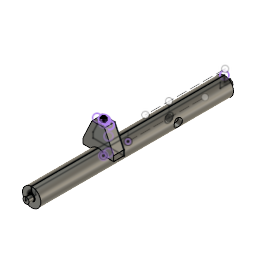
walek_2 (Autodesk Fusion 360 design; units mm, degrees)
part number: 2026-01-06-09-59-10-098
Autodesk Fusion 360 part; units mm, degrees
sketch "Szkic1" plane through (0, 0, 0) normal (1, 0, 0) x (0, 1, 0)
  line L0 (-99.5, 0) -> (-99.5, 3)
  line L1 (-99.5, 3) -> (-94.5, 3)
  line L2 (-94, 3.5) -> (-94, 9)
  line L3 (-94, 9) -> (94, 9)
  line L4 (94, 9) -> (94, 3.5)
  line L5 (94.5, 3) -> (99.5, 3)
  line L6 (99.5, 3) -> (99.5, 0)
  line L7 (0, 0) -> (0, 9) construction
  arc A0 (-94.5, 3) -> (-94, 3.5) centre (-94.5, 3.5) ccw
  arc A1 (94, 3.5) -> (94.5, 3) centre (94.5, 3.5) ccw
  line L8 (90, 0) -> (90, 5)
  line L9 (90, 5) -> (-90, 5)
  line L10 (-90, 5) -> (-90, 0)
  line L11 (99.5, 0) -> (90, 0)
  line L12 (-90, 0) -> (-99.5, 0)
  dimension "d1" = 199
  dimension "d3" = 5.5
  dimension "d4" = 9
  dimension "d5" = 3
  dimension "d6" = 3
  dimension "d7" = 5.5
  dimension "d9" = 0.5
  dimension "d10" = 0.5
  dimension "d11" = 4
  dimension "d12" = 4
  dimension "d13" = 4
  constraint vertical L0
  constraint perpendicular L0 L1
  constraint perpendicular L1 L2
  constraint perpendicular L2 L3
  constraint perpendicular L3 L4
  constraint perpendicular L4 L5
  constraint perpendicular L3 L6
  constraint perpendicular L0 L11
  constraint coincident L7.start origin
  constraint midpoint L3 L7.end
  constraint perpendicular L3 L7
  constraint coincident L7.start L11
  constraint tangent L1 A0
  constraint tangent L2 A0
  constraint tangent L5 A1
  constraint tangent L4 A1
  constraint vertical L8
  constraint horizontal L9
  constraint vertical L10
  constraint collinear L11 L12
  measures "d1" distance of L0 L6
  measures "d3" distance of L0 L2
  measures "d4" distance of L3 L11
  measures "d5" distance of L1 L11
  measures "d6" distance of L5 L11
  measures "d7" distance of L4 L6.end
  measures "d9" radius of A0
  measures "d10" radius of A1
  measures "d11" distance of L2 L10
  measures "d12" distance of L3 L9
  measures "d13" distance of L4 L8
revolve "Obrót1" add sketch "Szkic1" angle 360 about axis through (0, 99.5, 0) along (0, -1, 0)
sketch "Szkic2" plane through (0, 0, 0) normal (1, 0, 0) x (0, 1, 0)
  line L0 (94.6908, 14) -> (16.9684, 14) construction
  circle A0 centre (40, 0) radius 4
  line L1 (40, 14) -> (40, 0) construction
  line L2 (0, 0) -> (75, 0) construction
  point P0 (94, 9)
  dimension "d16" = 40
  dimension "d19" = 5
  dimension "d20" = 8
  constraint horizontal L0
  constraint coincident A0.centre L1.end
  constraint perpendicular L0 L1
  constraint coincident L2.start origin
  constraint perpendicular L1 L2
  constraint coincident A0.centre L2
  measures "d16" horizontal distance of L2.start L1.start
  measures "d19" vertical distance of L0.start P0
  measures "d20" diameter of A0
extrude "Wyciągnięcie proste2" cut sketch "Szkic2" along normal mid plane 60
ref_plane "Płaszczyzna konstrukcyjna1" through (0, -19, 0) normal (0, 1, 0) x (0, 0, 1)
sketch "Szkic4" plane through (0, -19, 0) normal (0, 1, 0) x (1, 0, 0)
  line L0 (-15, -5) -> (-15, -10)
  line L1 (-15, -10) -> (-6.1402, -29)
  line L2 (-6.1402, -29) -> (6.1402, -29)
  line L3 (6.1402, -29) -> (15, -10)
  line L4 (-15, -5) -> (15, -5)
  line L5 (15, -5) -> (15, -10)
  point P0 (0, -14)
  dimension "d43" = 5
  dimension "d46" = 155
  dimension "d48" = 30
  dimension "d49" = 15
  dimension "d51" = 5
  dimension "d52" = 155
  dimension "d53" = 5
  dimension "d54" = 24
  constraint perpendicular L0 L4
  constraint horizontal L4
  measures "d43" distance of L0.start L0.end
  measures "d46" angle of L0 L1
  measures "d48" distance of L0 L5
  measures "d49" distance of L5 P0
  measures "d51" distance of L4 origin
  measures "d52" angle of L3 L5
  measures "d53" distance of L3.end L4.end
  measures "d54" distance of L2 L4
extrude "Wyciągnięcie proste4" add sketch "Szkic4" against normal blind 10
ref_plane "Płaszczyzna konstrukcyjna2" through (0, -24, 17) normal (0, 1, 0) x (1, 0, 0)
sketch "Szkic5" plane through (0, -24, 0) normal (0, 1, 0) x (1, 0, 0)
  line L0 (0, -31.2) -> (0, -27.6)
  line L1 (6.1402, -29) -> (-6.1402, -29)
  arc A0 (2.245, -31.2) -> (0, -27.6) centre (0, -30.1) ccw
  line L2 (0, -31.2) -> (2.245, -31.2)
  dimension "d28" = 5
  dimension "d29" = 1.1
  dimension "d30" = 1.1
  constraint vertical L0
  constraint coincident A0.centre L0
  constraint coincident origin L0
  constraint perpendicular L0 L2
  measures "d28" diameter of A0
  measures "d29" distance of A0.centre L1
  measures "d30" distance of A0.centre L2
revolve "Obrót2" add sketch "Szkic5" angle 360 about axis through (0, -24, 31.2) along (0, 0, -1)
sketch "Szkic6" plane through (0, -24, 0) normal (0, 1, 0) x (1, 0, 0)
  arc A0 (2.245, -31.2) -> (0, -27.6) centre (0, -30.1) ccw
  line L0 (0, -31.85) -> (0, -28.35)
  arc A1 (0, -31.85) -> (0, -28.35) centre (0, -30.1) ccw
  dimension "d32" = 3.5
  constraint concentric A0 A1
  constraint vertical L0
  constraint coincident L0 origin
  measures "d32" diameter of A1
revolve "Obrót3" cut sketch "Szkic6" angle 360 about axis through (0, -24, 31.2) along (0, 0, -1)
sketch "Szkic7" plane through (0, -24, 0) normal (0, 1, 0) x (1, 0, 0)
  line L0 (-0.25, -29.7) -> (0.25, -29.7)
  line L1 (0.25, -29.7) -> (0.25, -31.2)
  line L2 (0.25, -31.2) -> (-0.25, -31.2)
  line L3 (-0.25, -31.2) -> (-0.25, -29.7)
  line L4 (0, -31.2) -> (2.245, -31.2)
  dimension "d34" = 0.5
  dimension "d35" = 1.5
  dimension "d36" = 0.25
  constraint horizontal L0
  constraint vertical L1
  constraint horizontal L2
  constraint vertical L3
  constraint coincident L1.end L4
  measures "d34" distance of L1.end L2.end
  measures "d35" distance of L0.end L1.end
  measures "d36" distance of L3 origin
extrude "Wyciągnięcie proste5" cut sketch "Szkic7" along normal blind 3
pattern_circular "Szyk kołowy1" count 4 over 360 about axis through (0, -24, 31.2) along (0, 0, -1) of "Wyciągnięcie proste5"
